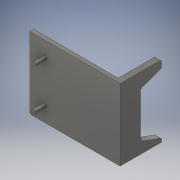
# Autodesk Inventor part: LucasCharles Part 10 final
Saved by Autodesk Inventor 2018 (Build 220112000, 112)
## iProperties
Created: 2018-05-19
Part Number: LucasCharles Part 10 final
Material: Stainless Steel, Austenitic
Document SubType Name: Modeling
Designer: Lucas
Density: 8 g/cm^3
Appearance: Semi-Polished
Author: Lucas
Autodesk Inventor part; units mm, degrees
ref_plane "YZ Plane" through (0, 0, 0) normal (1, 0, 0) x (0, 1, 0)
ref_plane "XZ Plane" through (0, 0, 0) normal (0, 1, 0) x (-1, 0, 0)
ref_plane "XY Plane" through (0, 0, 0) normal (0, 0, 1) x (1, 0, 0)
sketch "Sketch1" plane through (0, 0, 0) normal (0, 0, 1) x (1, 0, 0)
  line L0 (0, 0) -> (152.4, 0)
  line L1 (152.4, 0) -> (152.4, 120.65)
  line L2 (152.4, 120.65) -> (0, 120.65)
  line L3 (0, 120.65) -> (0, 0)
  dimension "d0" = 152.4
  dimension "d1" = 120.65
  constraints: 8 end point, 2 parallel, 1 horizontal, 1 perpendicular
  measures "d0" distance of L2.end L1.end
  measures "d1" distance between parallel lines of L0 L2
extrude "Extrusion1" add sketch "Sketch1" along normal blind 6.35
sketch "Sketch2" plane through (0, 0, 6.35) normal (0, 0, 1) x (1, 0, 0)
  line L0 (0, 0) -> (152.4, 0) projected
  line L1 (152.4, 120.65) -> (0, 120.65) projected
  line L2 (114.2866, 59.261) -> (0, 60.6355)
  line L3 (0, 120.65) -> (0, 0) projected
  line L4 (76.2, 0) -> (76.2, 120.65)
  circle A0 centre (25.4, 25.4) radius 3.175
  circle A1 centre (26.2401, 95.25) radius 3.175
  point P0 (114.7072, 94.0562)
  dimension "d18" = 25.4
  dimension "d20" = 25.4
  dimension "d23" = 25.4
  dimension "d24" = 26.2401
  dimension "d31" = 69.85
  dimension "d32" = 6.35
  constraints: 4 end point, 2 centre point, 2 midpoint, 1 point on line, 1 symmetric about line, 1 other
  measures "d18" distance from line of A0.centre L0
  measures "d20" distance from line of A0.centre L3
  measures "d23" distance from line of L1 A1.centre
  measures "d24" distance from line of L3 A1.centre
  measures "d31" vertical distance of A1.centre A0.centre
  measures "d32" diameter of A0
sketch "Sketch3" plane through (0, 0, 6.35) normal (0, 0, 1) x (1, 0, 0)
  point P0 (0, 0)
extrude "Extrusion4" add sketch "Sketch2" along normal blind 19.05 contours A0 | A1
thread "Thread5" size "3/8-16 UNC" class "2A" standard "ANSI Unified Screw Threads" full length
thread "Thread6" size "3/8-16 UNC" class "2A" standard "ANSI Unified Screw Threads" full length
sketch "Sketch7" plane through (0, 0, 0) normal (0, 0, -1) x (-1, 0, 0)
  line L0 (-152.4, 0) -> (-152.4, 120.65) projected
  line L1 (0, 0) -> (-152.4, 0) projected
  line L2 (-152.4, 120.65) -> (-142.875, 120.65)
  line L3 (-142.875, 120.65) -> (-142.875, 0)
  line L4 (-142.875, 0) -> (-152.4, 0)
  line L5 (-152.4, 0) -> (-152.4, 120.65)
  dimension "d36" = 9.525
  constraints: 8 end point, 2 parallel, 1 horizontal, 1 perpendicular, 1 point on line
  measures "d36" distance of L3.end L4.end
extrude "Extrusion6" add sketch "Sketch7" along normal blind 63.5
sketch "Sketch8" plane through (152.4, 0, 6.35) normal (1, 0, 0) x (0, 0, -1)
  line L0 (69.85, 0) -> (69.85, 120.65) projected
  line L1 (0, 0) -> (0, 120.65) projected
  line L2 (69.85, 107.95) -> (34.29, 95.5609)
  line L3 (34.29, 95.5609) -> (34.29, 19.05)
  line L4 (34.29, 19.05) -> (69.85, 6.35)
  point P0 (6.35, 0)
  point P1 (34.29, 108.2609)
  point P2 (34.29, 6.35)
  dimension "d39" = 12.7
  dimension "d40" = 12.7
  dimension "d41" = 34.29
  dimension "d42" = 34.29
  dimension "d43" = 34.29
  dimension "d44" = 34.29
  constraints: 6 end point, 2 point on line
  measures "d39" distance of L3.end point (34.29, 6.35)
  measures "d40" distance of L2.end point (34.29, 108.261)
  measures "d41" distance from line of L1 L2.end
  measures "d42" distance from line of L1 point (34.29, 108.261)
  measures "d43" distance from line of L1 L3.end
  measures "d44" distance from line of L1 point (34.29, 6.35)
extrude "Extrusion7" cut sketch "Sketch8" against normal blind 63.5
fillet "Fillet1" radius 3.175 5 edges at (147.6375, 120.65, -63.5) (147.6375, 107.95, -63.5) (147.6375, 95.5609, -27.94) (147.6375, 19.05, -27.94) (147.6375, 6.35, -63.5)
body "Solid1"
